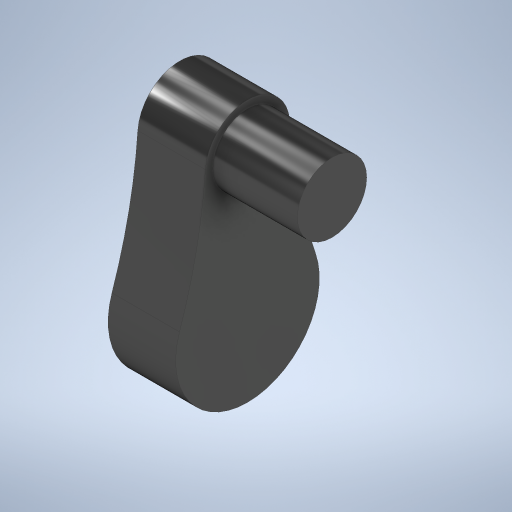
# Autodesk Inventor part: MotorAnkerNeu
Saved by Autodesk Inventor 2023 (Build 270158000, 158)
## iProperties
Created: 2024-02-23
Part Number: MotorAnkerNeu
Material: Generisch
Document SubType Name: Modeling
Designer: phili
Density: 1 g/cm^3
Appearance: Vorgabe
Author: phili
Autodesk Inventor part; units mm, degrees
ref_plane "YZ Plane" through (0, 0, 0) normal (1, 0, 0) x (0, 1, 0)
ref_plane "XZ Plane" through (0, 0, 0) normal (0, 1, 0) x (-1, 0, 0)
ref_plane "XY Plane" through (0, 0, 0) normal (0, 0, 1) x (1, 0, 0)
sketch "Skizze1" plane through (0, 0, 0) normal (1, 0, 0) x (0, 1, 0)
  circle A0 centre (7.8808, 0) radius 5
  circle A1 centre (-9.6192, 0) radius 8.5
  arc A2 (-6.8769, 8.0455) -> (8.2347, 4.9875) centre (12.4808, 64.837) ccw
  arc A3 (8.2347, -4.9875) -> (-6.8769, -8.0455) centre (12.4808, -64.837) ccw
  point P0 (0, 0)
  dimension "d0" = 10
  dimension "d1" = 17
  dimension "d2" = 17.5
  dimension "d3" = 60
  dimension "d4" = 0
  dimension "d5" = 0
  dimension "d6" = 60
  constraints: 8 point on circle, 4 centre point, 4 tangent
  measures "d0" diameter of A0
  measures "d1" diameter of A1
  measures "d2" distance of A1.centre A0.centre
  measures "d3" radius of A2
  measures "d4" vertical distance of point (0, 0) A0.centre
  measures "d5" vertical distance of point (0, 0) A1.centre
  measures "d6" radius of A3
extrude "Extrusion1" add sketch "Skizze1" along normal blind 8
sketch "Skizze2" plane through (8, 0, 0) normal (1, 0, 0) x (0, 0, -1)
  arc A0 (4.9875, 8.2347) -> (-4.9875, 8.2347) centre (0, 7.8808) ccw projected
  circle A1 centre (0, 7.8808) radius 4.1
  point P0 (0, 0)
  dimension "d9" = 8.2
  constraints: 1 centre point, 1 coincident
  measures "d9" diameter of A1
extrude "Extrusion2" add sketch "Skizze2" along normal blind 10
sketch "Skizze4" plane through (0, 0, 0) normal (-1, 0, 0) x (0, 0, 1)
  arc A0 (-8.0455, -6.8769) -> (8.0455, -6.8769) centre (0, -9.6192) ccw projected
  line L0 (-6.9859, -9.6192) -> (-3.493, -3.5692)
  line L1 (-3.493, -3.5692) -> (3.493, -3.5692)
  line L2 (3.493, -3.5692) -> (6.9859, -9.6192)
  line L3 (6.9859, -9.6192) -> (3.493, -15.6692)
  line L4 (3.493, -15.6692) -> (-3.493, -15.6692)
  line L5 (-3.493, -15.6692) -> (-6.9859, -9.6192)
  point P0 (0, 0)
  dimension "d15" = 12.1
  constraints: 12 end point, 1 coincident, 13 other
  measures "d15" distance between parallel lines of L3 L0
extrude "Extrusion4" cut sketch "Skizze4" against normal blind 6
